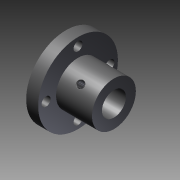
# Autodesk Inventor part: STHRBN12_ss
Saved by Autodesk Inventor 2016 (Build 200138000, 138)
## iProperties
Category: PARTsolutions
Company: MISUMI
Created: 2015-09-20
Part Number: STHRBN12_ss
Catalog Web Link: www.cadenas.de
Description: STHRBN, STHRN, SSTHRN, STHRNA, STHRND_SS-Shaft Supports - Bracket Shaped , Wide Holder - Standard Type - Round Flange
Vendor: MISUMI
Document SubType Name: Modeling
Designer: PARTuser1
Manufacturer: MISUMI
Mass: 11.2024 g
Surface Area: 54.6658 cm^2
Volume: 11.2024 cm^3
Density: 1 g/cm^3
Material: 一般
Appearance: PSOLRGB-192-192-192
PSOL_IDENT_0: {$CADENAS_DATA\23d-libs\misumi\metric\02_shaft_supports\sthrbn\sthrbn.prj},208 {VTYP=3D},{NB=STHRBN1
PSOL_IDENT_1: 2_ss},{LINA=STHRBN12},{NN=STHRBN, STHRN, SSTHRN, STHRNA, STHRND_SS},{DATE=21.05.2015 05:43:21},{GEOM
PSOL_IDENT_2: DATE=21.05.2015 05:43:21},{VERSION=},{LINEID=70},{LINESUBID=-1},{WBVAR=MAT,ST,M,ALT1}  {NB=STHRBN12_
PSOL_IDENT_3: ss},{LINA=STHRBN12},{KT=DUMMY},{PN=STHRBN12},{TYPE=STHRBN},{MAT=1018},{MATA= '1018', 'SS400 Equivale
PSOL_IDENT_4: nt',   '304', 'SUS304', '5056', 'A5056'  },{ST=Black Oxide},{ST0='Black Oxide','Black Oxide','Electr
PSOL_IDENT_5: oless Nickel Plating','Electroless Nickel Plating'},{D=12},{DTOL=+0.018/0},{DX=12},{N=5.0},{L=24},{D
PSOL_IDENT_6: 1=22},{H=40},{T=6},{LL=15},{M=M4},{MALG=},{M1=4},{M2=4},{M3=4},{M4='M4'},{P=32},{K=32},{W=25},{P1=28
PSOL_IDENT_7: },{F=16},{DD1=4.5},{DD11=4.5},{DD12=4.5},{ALT1=},{ALT1PN=},{MBM=0},{ML=0}
NN: STHRBN, STHRN, SSTHRN, STHRNA, STHRND_SS
NT: Shaft Supports - Bracket Shaped , Wide Holder - Standard Type - Round Flange
NB: STHRBN12_ss
NBSYN: $PN._ss
LINA: STHRBN12
PN: STHRBN12
MAT: SS400 Equivalent
ST: Black Oxide
D: 12
DTOL: +0.018/0
N: 5.0
L: 24
D1: 22
H: 40
T: 6
LL: 15
M: M4
P: 32
DD1: 4.5
ALT1: w/o MB (Hex Socket Set Screw Included)
MBM: 0
ML: 0
SUPPLIER: MISUMI
ARTICLENO: STHRBN12_ss
BOMINFO: STHRBN12
CREATOR: CADENAS GmbH
Title: STHRBN12
Author: Cadenas PARTsolutions
Comments: Shaft Supports - Bracket Shaped , Wide Holder - Standard Type - Round Flange
Autodesk Inventor part; units mm, degrees
ref_plane "YZ Plane" through (0, 0, 0) normal (1, 0, 0) x (0, 1, 0)
ref_plane "XZ Plane" through (0, 0, 0) normal (0, 1, 0) x (-1, 0, 0)
ref_plane "XY Plane" through (0, 0, 0) normal (0, 0, 1) x (1, 0, 0)
sketch "Sketch_1" plane through (0, 0, 0) normal (0, 0, 1) x (1, 0, 0)
  line L0 (24, 0) -> (0, 0)
  line L1 (0, 20) -> (0, 6)
  line L2 (0, 6) -> (24, 6)
  line L3 (24, 6) -> (24, 11)
  line L4 (24, 11) -> (6, 11)
  line L5 (6, 11) -> (6, 20)
  line L6 (6, 20) -> (0, 20)
  constraints: 14 end point
revolve "Revolution1" add sketch "Sketch_1" angle 360 about axis through (24, 0, 0) along (1, 0, 0)
sketch "Sketch2" plane through (0, 0, 0) normal (-1, 0, 0) x (0, 0, 1)
  point P0 (0, 16)
hole "Hole1" at (0, 16, 0) direction (1, 0, 0) diameter 4.5 depth 6
pattern_linear "Rectangular Pattern1" count 2 spacing 22.6274 along (0, -0.7071, 0.7071) count 2 spacing 22.6274 along (0, -0.7071, -0.7071) of "Hole1"
sketch "Sketch_4" plane through (15, 0, 0) normal (1, 0, 0) x (0, 0, -1)
  line L0 (-7.7782, -7.7782) -> (-3.5355, -3.5355)
  line L1 (-3.5355, -3.5355) -> (-2.3893, -4.6818)
  line L2 (-2.3893, -4.6818) -> (-6.364, -8.6564)
  line L3 (-6.364, -8.6564) -> (-6.364, -9.1924)
  line L4 (-6.364, -9.1924) -> (-7.7782, -7.7782)
  line L5 (-7.7782, -7.7782) -> (-3.5355, -3.5355)
  constraints: 12 end point
revolve "Revolution2" cut sketch "Sketch_4" angle 360 about axis through (15, -7.7782, 7.7782) along (0, -0.7071, 0.7071)
thread "Thread1" size "M4x0.7" class "6H" standard "ISO Metric profile" full length
sketch "Sketch_5" plane through (15, 0, 0) normal (1, 0, 0) x (0, 0, -1)
  line L0 (-7.7782, 7.7782) -> (-3.5355, 3.5355)
  line L1 (-3.5355, 3.5355) -> (-4.6818, 2.3893)
  line L2 (-4.6818, 2.3893) -> (-8.6564, 6.364)
  line L3 (-8.6564, 6.364) -> (-9.1924, 6.364)
  line L4 (-9.1924, 6.364) -> (-7.7782, 7.7782)
  line L5 (-7.7782, 7.7782) -> (-3.5355, 3.5355)
  constraints: 12 end point
revolve "Revolution3" cut sketch "Sketch_5" angle 360 about axis through (15, 7.7782, 7.7782) along (0, 0.7071, 0.7071)
thread "Thread2" size "M4x0.7" class "6H" standard "ISO Metric profile" full length
body "Solid1"
